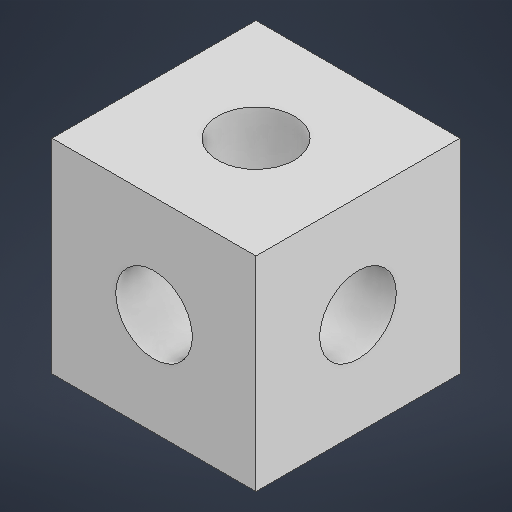
# Autodesk Inventor part: 8X
Saved by Autodesk Inventor 2025 (Build 290162000, 162)
## iProperties
Created: 2026-04-21
Part Number: 8X
Material: 常规
Document SubType Name: Modeling
Designer: XH
Density: 1 g/cm^3
Appearance: 默认
Author: XH
Autodesk Inventor part; units mm, degrees
ref_plane "YZ Plane" through (0, 0, 0) normal (1, 0, 0) x (0, 1, 0)
ref_plane "XZ Plane" through (0, 0, 0) normal (0, 1, 0) x (-1, 0, 0)
ref_plane "XY Plane" through (0, 0, 0) normal (0, 0, 1) x (1, 0, 0)
sketch "草图1" plane through (0, 0, 0) normal (0, 0, 1) x (1, 0, 0)
  line L0 (4, -4) -> (-4, -4)
  line L1 (-4, -4) -> (-4, 4)
  line L2 (-4, 4) -> (4, 4)
  line L3 (4, 4) -> (4, -4)
  line L4 (4, -4) -> (-4, 4) construction
  line L5 (-4, -4) -> (4, 4) construction
  point P0 (0, 0)
  dimension "d0" = 8
  dimension "d1" = 8
  constraints: 12 end point, 2 midpoint, 2 parallel, 1 horizontal, 1 perpendicular
  measures "d0" distance of L1.end L2.end
  measures "d1" distance of L2.end L0.start
extrude "拉伸1" add sketch "草图1" along normal blind 8
sketch "草图2" plane through (-4, -4, 0) normal (0, -1, 0) x (1, 0, 0)
  line L0 (8, 8) -> (0, 8) projected
  line L1 (0, 8) -> (8, 0)
  circle A0 centre (4, 4) radius 1.5
  point P0 (4, 0)
  dimension "d4" = 3
  constraints: 2 end point, 1 centre point, 1 midpoint
  measures "d4" diameter of A0
extrude "拉伸2" cut sketch "草图2" against normal blind 8
sketch "草图3" plane through (0, 0, 0) normal (0, 0, -1) x (-1, 0, 0)
  circle A0 centre (0, 0) radius 1.5
  dimension "d7" = 3
  constraints: 1 centre point, 1 coincident
  measures "d7" diameter of A0
extrude "拉伸3" cut sketch "草图3" against normal blind 8
sketch "草图4" plane through (4, -4, 0) normal (1, 0, 0) x (0, 0, -1)
  line L0 (0, 8) -> (0, 0) projected
  line L1 (0, 8) -> (-8, 0)
  circle A0 centre (-4, 4) radius 1.5
  point P0 (0, 4)
  dimension "d10" = 3
  constraints: 2 end point, 1 centre point, 1 coincident, 1 midpoint
  measures "d10" diameter of A0
extrude "拉伸4" cut sketch "草图4" against normal blind 14.25
